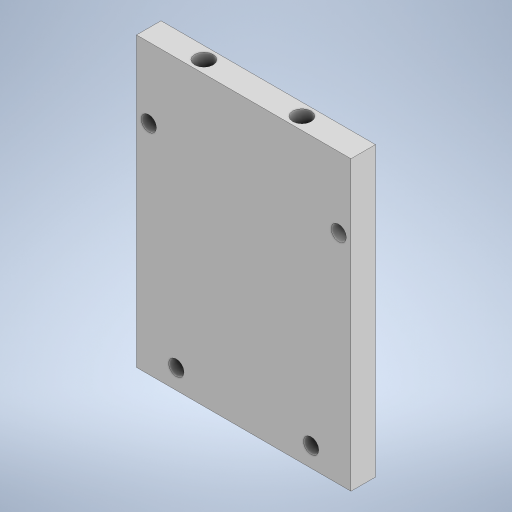
# Autodesk Inventor part: Suportmotor
Saved by Autodesk Inventor 2023 (Build 270158000, 158)
## iProperties
Created: 2022-09-23
Part Number: Suportmotor
Material: Generic
Document SubType Name: Modelado
Designer: hiago.sodre
Density: 1 g/cm^3
Appearance: Default
Sheet Metal Rule: Por defecto_mm
Author: hiago.sodre
Autodesk Inventor part; units mm, degrees
ref_plane "YZ Plane" through (0, 0, 0) normal (1, 0, 0) x (0, 1, 0)
ref_plane "XZ Plane" through (0, 0, 0) normal (0, 1, 0) x (-1, 0, 0)
ref_plane "XY Plane" through (0, 0, 0) normal (0, 0, 1) x (1, 0, 0)
sketch "Sketch12" plane through (0, 0, 0) normal (0, 0, 1) x (1, 0, 0)
  line L0 (0, 0) -> (35, 0)
  line L1 (35, 0) -> (35, 47)
  line L2 (35, 47) -> (0, 47)
  line L3 (0, 47) -> (0, 0)
  line L4 (0, 47) -> (2, 47) construction
  line L5 (2, 47) -> (2, 35.5) construction
  line L6 (35, 47) -> (33, 47) construction
  line L7 (33, 47) -> (33, 35.5) construction
  circle A0 centre (33, 35.5) radius 1.25
  circle A1 centre (2, 35.5) radius 1.25
  line L8 (0, 0) -> (6.5, 0) construction
  line L9 (35, 0) -> (28.5, 0) construction
  line L10 (6.5, 0) -> (6.5, 3.2) construction
  line L11 (28.5, 0) -> (28.5, 3.2) construction
  circle A2 centre (6.5, 3.2) radius 1.25
  circle A3 centre (28.5, 3.2) radius 1.25
  dimension "d49" = 35
  dimension "d50" = 47
  dimension "d97" = 2
  dimension "d98" = 11.5
  dimension "d99" = 2
  dimension "d100" = 2.5
  dimension "d101" = 2.5
  dimension "d102" = 11.5
  dimension "d103" = 6.5
  dimension "d104" = 6.5
  dimension "d105" = 3.2
  dimension "d106" = 3.2
  dimension "d107" = 2.5
  dimension "d108" = 2.5
  constraints: 24 end point, 4 centre point, 4 coincident, 4 point on line, 3 perpendicular, 2 parallel, 2 vertical, 1 horizontal
  measures "d49" distance of L2.end L1.end
  measures "d50" distance of L1.end L0.end
  measures "d97" distance of L2.end L4.end
  measures "d98" distance of L4.end L5.end
  measures "d99" distance of L1.end L6.end
  measures "d100" diameter of A0
  measures "d101" diameter of A1
  measures "d102" distance of L6.end L7.end
  measures "d103" distance of L0.start L8.end
  measures "d104" distance of L0.end L9.end
  measures "d105" distance of L8.end L10.end
  measures "d106" distance of L9.end L11.end
  measures "d107" diameter of A2
  measures "d108" diameter of A3
extrude "Extrusión8" add sketch "Sketch12" along normal blind 4
sketch "Boceto21" plane through (0, 0, 0) normal (0, -1, 0) x (1, 0, 0)
  line L0 (35, 0) -> (35, 4) construction
  line L1 (35, 0) -> (35, 4) construction
  line L2 (0, 0) -> (0, 4) construction
  line L3 (0, 0) -> (0, 4) construction
  line L4 (0, 2) -> (35, 2) construction
  line L5 (35, 2) -> (25, 2) construction
  line L6 (0, 2) -> (9, 2) construction
  circle A0 centre (9, 2) radius 1.5
  circle A1 centre (25, 2) radius 1.5
  dimension "d111" = 10
  dimension "d112" = 9
  dimension "d113" = 3
  dimension "d114" = 3
  constraints: 10 end point, 2 centre point, 2 coincident, 2 collinear, 2 midpoint, 2 point on line
  measures "d111" distance of L4.end L5.end
  measures "d112" distance of L4.start L6.end
  measures "d113" diameter of A0
  measures "d114" diameter of A1
extrude "Extrusión9" cut sketch "Boceto21" along normal through all both and the other way through all
equation "\"BendRadius\" = Thickness"
equation "\"BendReliefWidth\" = Thickness"
equation "\"BendReliefDepth\" = 0.5 * Thickness"
equation "\"CornerReliefSize\" = 4 * Thickness"
equation "\"MinimumRemnant\" = 2 * Thickness"
equation "\"TransitionRadius\" = BendRadius"
equation "\"JacobiRadiusSize\" = BendRadius"
equation "\"GapSize\" = Thickness"
equation "\"Thickness\" = 1"
